Autodesk Inventor part; units mm, degrees
(part 2 of 3)
  line L292 (-4.8745, -39.6988) -> (-5.1074, -39.4176)
  spline S165 degree 2 poles (-5.1074, -39.4176) (-4.9285, -39.2301) (-4.4598, -39) (-4.1502, -39) knots 0 0 0 1 2 2 2
  spline S166 degree 2 poles (-4.1502, -39) (-3.94, -39) (-3.5906, -39.125) (-3.3406, -39.3636) (-3.2014, -39.7073) (-3.2014, -39.9232) knots 0 0 0 1 2 3 4 4 4
  spline S167 degree 2 poles (-3.2014, -39.9232) (-3.2014, -40.1078) (-3.298, -40.4174) (-3.494, -40.7242) (-3.7923, -41.0537) (-3.9968, -41.2525) knots 0 0 0 1 2 3 4 4 4
  line L293 (-3.9968, -41.2525) -> (-4.5706, -41.8121)
  line L294 (-4.5706, -41.8121) -> (-3.031, -41.8121)
  line L295 (-3.031, -41.8121) -> (-3.031, -42.2154)
  spline S168 degree 2 poles (-0.2274, -40.6304) (-0.2274, -40.994) (-0.3723, -41.5934) (-0.6677, -42.0223) (-1.108, -42.2581) (-1.4034, -42.2581) knots 0 0 0 1 2 3 4 4 4
  spline S169 degree 2 poles (-1.4034, -42.2581) (-1.659, -42.2581) (-2.0738, -42.0677) (-2.372, -41.6672) (-2.5311, -41.0537) (-2.5311, -40.6304) knots 0 0 0 1 2 3 4 4 4
  spline S170 degree 2 poles (-2.5311, -40.6304) (-2.5311, -40.2669) (-2.3834, -39.6647) (-2.0908, -39.2358) (-1.6477, -39) (-1.3551, -39) knots 0 0 0 1 2 3 4 4 4
  spline S171 degree 2 poles (-1.3551, -39) (-1.0995, -39) (-0.6819, -39.1903) (-0.3865, -39.5908) (-0.2274, -40.2072) (-0.2274, -40.6304) knots 0 0 0 1 2 3 4 4 4
  spline S172 degree 2 poles (-0.6535, -40.6447) (-0.6535, -40.5623) (-0.6649, -40.4004) (-0.6734, -40.3237) knots 0 0 0 1 2 2 2
  line L296 (-0.6734, -40.3237) -> (-2.0141, -41.3178)
  spline S173 degree 2 poles (-2.0141, -41.3178) (-1.98, -41.4457) (-1.8664, -41.6587) (-1.7102, -41.8121) (-1.5085, -41.8973) (-1.3778, -41.8973) knots 0 0 0 1 2 3 4 4 4
  spline S174 degree 2 poles (-1.3778, -41.8973) (-1.2131, -41.8973) (-0.9461, -41.7382) (-0.7558, -41.4201) (-0.6535, -40.9514) (-0.6535, -40.6447) knots 0 0 0 1 2 3 4 4 4
  spline S175 degree 2 poles (-2.105, -40.6162) (-2.105, -40.6901) (-2.1022, -40.8406) (-2.0965, -40.9117) knots 0 0 0 1 2 2 2
  line L297 (-2.0965, -40.9117) -> (-0.7529, -39.9203)
  spline S176 degree 2 poles (-0.7529, -39.9203) (-0.7899, -39.7953) (-0.9006, -39.5908) (-1.0569, -39.4431) (-1.2557, -39.3607) (-1.3778, -39.3607) knots 0 0 0 1 2 3 4 4 4
  spline S177 degree 2 poles (-1.3778, -39.3607) (-1.5454, -39.3607) (-1.8124, -39.5198) (-2.0028, -39.8379) (-2.105, -40.3066) (-2.105, -40.6162) knots 0 0 0 1 2 3 4 4 4
  line L298 (2.116, -42.2154) -> (2.116, -40.4657)
  spline S178 degree 2 poles (2.116, -40.4657) (2.116, -40.3521) (2.0989, -40.2072) (2.0648, -40.122) (2.0137, -40.0879) (1.974, -40.0879) knots 0 0 0 1 2 3 4 4 4
  spline S179 degree 2 poles (1.974, -40.0879) (1.9285, -40.0879) (1.8518, -40.1447) (1.7638, -40.2782) (1.6587, -40.4941) (1.5848, -40.6503) knots 0 0 0 1 2 3 4 4 4
  line L299 (1.5848, -40.6503) -> (1.5848, -42.2154)
  line L300 (1.5848, -42.2154) -> (1.1616, -42.2154)
  line L301 (1.1616, -42.2154) -> (1.1616, -40.5111)
  spline S180 degree 2 poles (1.1616, -40.5111) (1.1616, -40.3776) (1.1445, -40.2129) (1.1104, -40.122) (1.0565, -40.0879) (1.0167, -40.0879) knots 0 0 0 1 2 3 4 4 4
  spline S181 degree 2 poles (1.0167, -40.0879) (0.9769, -40.0879) (0.9031, -40.1362) (0.815, -40.2612) (0.7042, -40.4799) (0.6304, -40.6503) knots 0 0 0 1 2 3 4 4 4
  line L302 (0.6304, -40.6503) -> (0.6304, -42.2154)
  line L303 (0.6304, -42.2154) -> (0.2072, -42.2154)
  line L304 (0.2072, -42.2154) -> (0.2072, -39.7811)
  line L305 (0.2072, -39.7811) -> (0.5594, -39.7811)
  line L306 (0.5594, -39.7811) -> (0.5793, -40.2441)
  spline S182 degree 2 poles (0.5793, -40.2441) (0.6446, -40.105) (0.7639, -39.9118) (0.8889, -39.7925) (1.0337, -39.7357) (1.119, -39.7357) knots 0 0 0 1 2 3 4 4 4
  spline S183 degree 2 poles (1.119, -39.7357) (1.3178, -39.7357) (1.5223, -39.9942) (1.5223, -40.264) knots 0 0 0 1 2 2 2
  spline S184 degree 2 poles (1.5223, -40.264) (1.5791, -40.1362) (1.6927, -39.9402) (1.8206, -39.8067) (1.9768, -39.7357) (2.0791, -39.7357) knots 0 0 0 1 2 3 4 4 4
  spline S185 degree 2 poles (2.0791, -39.7357) (2.5392, -39.7357) (2.5392, -40.443) knots 0 0 0 1 1 1
  line L307 (2.5392, -40.443) -> (2.5392, -42.2154)
  line L308 (2.5392, -42.2154) -> (2.116, -42.2154)
  line L309 (5.4308, -42.2154) -> (4.9593, -42.2154)
  line L310 (4.9593, -42.2154) -> (4.7406, -41.5252)
  line L311 (4.7406, -41.5252) -> (3.4141, -41.5252)
  line L312 (3.4141, -41.5252) -> (3.1925, -42.2154)
  line L313 (3.1925, -42.2154) -> (2.7466, -42.2154)
  line L314 (2.7466, -42.2154) -> (3.7976, -39.0454)
  line L315 (3.7976, -39.0454) -> (4.3912, -39.0454)
  line L316 (4.3912, -39.0454) -> (5.4308, -42.2154)
  line L317 (4.6156, -41.1389) -> (4.0788, -39.4403)
  line L318 (4.0788, -39.4403) -> (3.5362, -41.1389)
  line L319 (3.5362, -41.1389) -> (4.6156, -41.1389)
  line L320 (-112.276, -39.2585) -> (-113.3553, -42.4285)
  line L321 (-113.3553, -42.4285) -> (-113.9377, -42.4285)
  line L322 (-113.9377, -42.4285) -> (-114.9886, -39.2585)
  line L323 (-114.9886, -39.2585) -> (-114.5029, -39.2585)
  line L324 (-114.5029, -39.2585) -> (-113.8184, -41.3945)
  line L325 (-113.8184, -41.3945) -> (-113.6224, -42.0223)
  line L326 (-113.6224, -42.0223) -> (-113.4235, -41.3945)
  line L327 (-113.4235, -41.3945) -> (-112.739, -39.2585)
  line L328 (-112.739, -39.2585) -> (-112.276, -39.2585)
  spline S186 degree 2 poles (-109.7593, -41.19) (-109.7593, -41.4741) (-109.9183, -41.9484) (-110.2194, -42.2836) (-110.6512, -42.4711) (-110.9267, -42.4711) knots 0 0 0 1 2 3 4 4 4
  spline S187 degree 2 poles (-110.9267, -42.4711) (-111.188, -42.4711) (-111.6028, -42.3092) (-111.8897, -41.9939) (-112.043, -41.528) (-112.043, -41.2241) knots 0 0 0 1 2 3 4 4 4
  spline S188 degree 2 poles (-112.043, -41.2241) (-112.043, -40.9401) (-111.884, -40.4714) (-111.5829, -40.1362) (-111.1511, -39.9487) (-110.8756, -39.9487) knots 0 0 0 1 2 3 4 4 4
  spline S189 degree 2 poles (-110.8756, -39.9487) (-110.6143, -39.9487) (-110.1996, -40.1106) (-109.9127, -40.4231) (-109.7593, -40.8889) (-109.7593, -41.19) knots 0 0 0 1 2 3 4 4 4
  spline S190 degree 2 poles (-110.191, -41.2099) (-110.191, -40.9827) (-110.2904, -40.6475) (-110.4751, -40.4203) (-110.7392, -40.3066) (-110.9012, -40.3066) knots 0 0 0 1 2 3 4 4 4
  spline S191 degree 2 poles (-110.9012, -40.3066) (-111.0915, -40.3066) (-111.3585, -40.4543) (-111.5317, -40.7015) (-111.6113, -41.0281) (-111.6113, -41.2099) knots 0 0 0 1 2 3 4 4 4
  spline S192 degree 2 poles (-111.6113, -41.2099) (-111.6113, -41.4343) (-111.5119, -41.7723) (-111.3272, -41.9996) (-111.0659, -42.1132) (-110.9012, -42.1132) knots 0 0 0 1 2 3 4 4 4
  spline S193 degree 2 poles (-110.9012, -42.1132) (-110.7108, -42.1132) (-110.4438, -41.9655) (-110.2706, -41.7184) (-110.191, -41.3917) (-110.191, -41.2099) knots 0 0 0 1 2 3 4 4 4
  line L329 (-108.3163, -39.3465) -> (-109.0378, -39.3465)
  line L330 (-109.0378, -39.3465) -> (-109.0378, -39)
  line L331 (-109.0378, -39) -> (-107.8902, -39)
  line L332 (-107.8902, -39) -> (-107.8902, -42.0763)
  line L333 (-107.8902, -42.0763) -> (-107.1659, -42.0763)
  line L334 (-107.1659, -42.0763) -> (-107.1659, -42.4285)
  line L335 (-107.1659, -42.4285) -> (-109.1173, -42.4285)
  line L336 (-109.1173, -42.4285) -> (-109.1173, -42.0763)
  line L337 (-109.1173, -42.0763) -> (-108.3163, -42.0763)
  line L338 (-108.3163, -42.0763) -> (-108.3163, -39.3465)
  spline S194 degree 2 poles (-104.4504, -42.3944) (-104.5924, -42.4313) (-104.8992, -42.4626) (-105.0582, -42.4626) knots 0 0 0 1 2 2 2
  spline S195 degree 2 poles (-105.0582, -42.4626) (-105.5156, -42.4626) (-105.9672, -42.0479) (-105.9672, -41.6189) knots 0 0 0 1 2 2 2
  line L339 (-105.9672, -41.6189) -> (-105.9672, -40.3492)
  line L340 (-105.9672, -40.3492) -> (-106.6489, -40.3492)
  line L341 (-106.6489, -40.3492) -> (-106.6489, -39.9942)
  line L342 (-106.6489, -39.9942) -> (-105.9672, -39.9942)
  line L343 (-105.9672, -39.9942) -> (-105.9672, -39.3238)
  line L344 (-105.9672, -39.3238) -> (-105.544, -39.2159)
  line L345 (-105.544, -39.2159) -> (-105.544, -39.9942)
  line L346 (-105.544, -39.9942) -> (-104.4504, -39.9942)
  line L347 (-104.4504, -39.9942) -> (-104.4504, -40.3492)
  line L348 (-104.4504, -40.3492) -> (-105.544, -40.3492)
  line L349 (-105.544, -40.3492) -> (-105.544, -41.5849)
  spline S196 degree 2 poles (-105.544, -41.5849) (-105.544, -41.8462) (-105.2656, -42.1047) (-104.9929, -42.1047) knots 0 0 0 1 2 2 2
  spline S197 degree 2 poles (-104.9929, -42.1047) (-104.8765, -42.1047) (-104.6009, -42.0677) (-104.4504, -42.0308) knots 0 0 0 1 2 2 2
  line L350 (-104.4504, -42.0308) -> (-104.4504, -42.3944)
  line L351 (-101.9422, -42.4285) -> (-101.9422, -40.6787)
  spline S198 degree 2 poles (-101.9422, -40.6787) (-101.9422, -40.5651) (-101.9593, -40.4203) (-101.9933, -40.335) (-102.0445, -40.3009) (-102.0842, -40.3009) knots 0 0 0 1 2 3 4 4 4
  spline S199 degree 2 poles (-102.0842, -40.3009) (-102.1297, -40.3009) (-102.2064, -40.3578) (-102.2944, -40.4913) (-102.3995, -40.7071) (-102.4734, -40.8634) knots 0 0 0 1 2 3 4 4 4
  line L352 (-102.4734, -40.8634) -> (-102.4734, -42.4285)
  line L353 (-102.4734, -42.4285) -> (-102.8966, -42.4285)
  line L354 (-102.8966, -42.4285) -> (-102.8966, -40.7242)
  spline S200 degree 2 poles (-102.8966, -40.7242) (-102.8966, -40.5907) (-102.9137, -40.4259) (-102.9478, -40.335) (-103.0017, -40.3009) (-103.0415, -40.3009) knots 0 0 0 1 2 3 4 4 4
  spline S201 degree 2 poles (-103.0415, -40.3009) (-103.0813, -40.3009) (-103.1551, -40.3492) (-103.2432, -40.4742) (-103.3539, -40.6929) (-103.4278, -40.8634) knots 0 0 0 1 2 3 4 4 4
  line L355 (-103.4278, -40.8634) -> (-103.4278, -42.4285)
  line L356 (-103.4278, -42.4285) -> (-103.851, -42.4285)
  line L357 (-103.851, -42.4285) -> (-103.851, -39.9942)
  line L358 (-103.851, -39.9942) -> (-103.4988, -39.9942)
  line L359 (-103.4988, -39.9942) -> (-103.4789, -40.4572)
  spline S202 degree 2 poles (-103.4789, -40.4572) (-103.4136, -40.318) (-103.2943, -40.1248) (-103.1693, -40.0055) (-103.0244, -39.9487) (-102.9392, -39.9487) knots 0 0 0 1 2 3 4 4 4
  spline S203 degree 2 poles (-102.9392, -39.9487) (-102.7404, -39.9487) (-102.5359, -40.2072) (-102.5359, -40.4771) knots 0 0 0 1 2 2 2
  spline S204 degree 2 poles (-102.5359, -40.4771) (-102.4791, -40.3492) (-102.3654, -40.1532) (-102.2376, -40.0197) (-102.0814, -39.9487) (-101.9791, -39.9487) knots 0 0 0 1 2 3 4 4 4
  spline S205 degree 2 poles (-101.9791, -39.9487) (-101.519, -39.9487) (-101.519, -40.656) knots 0 0 0 1 1 1
  line L360 (-101.519, -40.656) -> (-101.519, -42.4285)
  line L361 (-101.519, -42.4285) -> (-101.9422, -42.4285)
  spline S206 degree 2 poles (-98.8915, -41.0821) (-98.8915, -41.1701) (-98.8972, -41.2923) (-98.9, -41.3463) knots 0 0 0 1 2 2 2
  line L362 (-98.9, -41.3463) -> (-100.6129, -41.3463)
  spline S207 degree 2 poles (-100.6129, -41.3463) (-100.6129, -41.7184) (-100.1953, -42.1189) (-99.8005, -42.1189) knots 0 0 0 1 2 2 2
  spline S208 degree 2 poles (-99.8005, -42.1189) (-99.6954, -42.1189) (-99.4823, -42.1018) (-99.2807, -42.0734) (-99.0989, -42.0365) (-99.0222, -42.0138) knots 0 0 0 1 2 3 4 4 4
  line L363 (-99.0222, -42.0138) -> (-99.0222, -42.3603)
  spline S209 degree 2 poles (-99.0222, -42.3603) (-99.1954, -42.4086) (-99.63, -42.4711) (-99.863, -42.4711) knots 0 0 0 1 2 2 2
  spline S210 degree 2 poles (-99.863, -42.4711) (-100.1754, -42.4711) (-100.6271, -42.3007) (-100.914, -41.9797) (-101.0531, -41.511) (-101.0531, -41.2156) knots 0 0 0 1 2 3 4 4 4
  spline S211 degree 2 poles (-101.0531, -41.2156) (-101.0531, -40.9571) (-100.9054, -40.4998) (-100.6214, -40.1532) (-100.2095, -39.9487) (-99.9482, -39.9487) knots 0 0 0 1 2 3 4 4 4
  spline S212 degree 2 poles (-99.9482, -39.9487) (-99.6925, -39.9487) (-99.2977, -40.1078) (-99.0307, -40.4032) (-98.8915, -40.8208) (-98.8915, -41.0821) knots 0 0 0 1 2 3 4 4 4
  spline S213 degree 2 poles (-99.3318, -41.0224) (-99.3233, -40.8605) (-99.4028, -40.5907) (-99.5647, -40.3947) (-99.8062, -40.2867) (-99.9681, -40.2867) knots 0 0 0 1 2 3 4 4 4
  spline S214 degree 2 poles (-99.9681, -40.2867) (-100.1044, -40.2867) (-100.3345, -40.3947) (-100.4992, -40.5878) (-100.6015, -40.8605) (-100.6129, -41.0224) knots 0 0 0 1 2 3 4 4 4
  line L364 (-100.6129, -41.0224) -> (-99.3318, -41.0224)
  spline S215 degree 2 poles (-96.2527, -42.3944) (-96.3947, -42.4313) (-96.7015, -42.4626) (-96.8606, -42.4626) knots 0 0 0 1 2 2 2
  spline S216 degree 2 poles (-96.8606, -42.4626) (-97.3179, -42.4626) (-97.7695, -42.0479) (-97.7695, -41.6189) knots 0 0 0 1 2 2 2
  line L365 (-97.7695, -41.6189) -> (-97.7695, -40.3492)
  line L366 (-97.7695, -40.3492) -> (-98.4512, -40.3492)
  line L367 (-98.4512, -40.3492) -> (-98.4512, -39.9942)
  line L368 (-98.4512, -39.9942) -> (-97.7695, -39.9942)
  line L369 (-97.7695, -39.9942) -> (-97.7695, -39.3238)
  line L370 (-97.7695, -39.3238) -> (-97.3463, -39.2159)
  line L371 (-97.3463, -39.2159) -> (-97.3463, -39.9942)
  line L372 (-97.3463, -39.9942) -> (-96.2527, -39.9942)
  line L373 (-96.2527, -39.9942) -> (-96.2527, -40.3492)
  line L374 (-96.2527, -40.3492) -> (-97.3463, -40.3492)
  line L375 (-97.3463, -40.3492) -> (-97.3463, -41.5849)
  spline S217 degree 2 poles (-97.3463, -41.5849) (-97.3463, -41.8462) (-97.0679, -42.1047) (-96.7952, -42.1047) knots 0 0 0 1 2 2 2
  spline S218 degree 2 poles (-96.7952, -42.1047) (-96.6788, -42.1047) (-96.4032, -42.0677) (-96.2527, -42.0308) knots 0 0 0 1 2 2 2
  line L376 (-96.2527, -42.0308) -> (-96.2527, -42.3944)
  spline S219 degree 2 poles (-93.4264, -41.0821) (-93.4264, -41.1701) (-93.4321, -41.2923) (-93.4349, -41.3463) knots 0 0 0 1 2 2 2
  line L377 (-93.4349, -41.3463) -> (-95.1477, -41.3463)
  spline S220 degree 2 poles (-95.1477, -41.3463) (-95.1477, -41.7184) (-94.7302, -42.1189) (-94.3353, -42.1189) knots 0 0 0 1 2 2 2
  spline S221 degree 2 poles (-94.3353, -42.1189) (-94.2303, -42.1189) (-94.0172, -42.1018) (-93.8155, -42.0734) (-93.6337, -42.0365) (-93.5571, -42.0138) knots 0 0 0 1 2 3 4 4 4
  line L378 (-93.5571, -42.0138) -> (-93.5571, -42.3603)
  spline S222 degree 2 poles (-93.5571, -42.3603) (-93.7303, -42.4086) (-94.1649, -42.4711) (-94.3978, -42.4711) knots 0 0 0 1 2 2 2
  spline S223 degree 2 poles (-94.3978, -42.4711) (-94.7103, -42.4711) (-95.1619, -42.3007) (-95.4488, -41.9797) (-95.588, -41.511) (-95.588, -41.2156) knots 0 0 0 1 2 3 4 4 4
  spline S224 degree 2 poles (-95.588, -41.2156) (-95.588, -40.9571) (-95.4403, -40.4998) (-95.1563, -40.1532) (-94.7444, -39.9487) (-94.4831, -39.9487) knots 0 0 0 1 2 3 4 4 4
  spline S225 degree 2 poles (-94.4831, -39.9487) (-94.2274, -39.9487) (-93.8326, -40.1078) (-93.5656, -40.4032) (-93.4264, -40.8208) (-93.4264, -41.0821) knots 0 0 0 1 2 3 4 4 4
  spline S226 degree 2 poles (-93.8667, -41.0224) (-93.8581, -40.8605) (-93.9377, -40.5907) (-94.0996, -40.3947) (-94.341, -40.2867) (-94.5029, -40.2867) knots 0 0 0 1 2 3 4 4 4
  spline S227 degree 2 poles (-94.5029, -40.2867) (-94.6393, -40.2867) (-94.8694, -40.3947) (-95.0341, -40.5878) (-95.1364, -40.8605) (-95.1477, -41.0224) knots 0 0 0 1 2 3 4 4 4
  line L379 (-95.1477, -41.0224) -> (-93.8667, -41.0224)
  line L380 (-92.6509, -39.9942) -> (-92.2646, -39.9942)
  line L381 (-92.2646, -39.9942) -> (-92.2533, -40.443)
  spline S228 degree 2 poles (-92.2533, -40.443) (-92.0374, -40.1816) (-91.6198, -39.9487) (-91.404, -39.9487) knots 0 0 0 1 2 2 2
  spline S229 degree 2 poles (-91.404, -39.9487) (-91.0262, -39.9487) (-90.637, -40.4401) (-90.6512, -40.923) knots 0 0 0 1 2 2 2
  line L382 (-90.6512, -40.923) -> (-91.0773, -40.923)
  spline S230 degree 2 poles (-91.0773, -40.923) (-91.0688, -40.602) (-91.2704, -40.3123) (-91.4664, -40.3123) knots 0 0 0 1 2 2 2
  spline S231 degree 2 poles (-91.4664, -40.3123) (-91.5517, -40.3123) (-91.7221, -40.372) (-91.9039, -40.5083) (-92.1084, -40.7157) (-92.2249, -40.8662) knots 0 0 0 1 2 3 4 4 4
  line L383 (-92.2249, -40.8662) -> (-92.2249, -42.4285)
  line L384 (-92.2249, -42.4285) -> (-92.6509, -42.4285)
  line L385 (-92.6509, -42.4285) -> (-92.6509, -39.9942)
  spline S232 degree 2 poles (-85.1577, -40.8435) (-85.1577, -41.2071) (-85.3026, -41.8064) (-85.598, -42.2353) (-86.0382, -42.4711) (-86.3337, -42.4711) knots 0 0 0 1 2 3 4 4 4
  spline S233 degree 2 poles (-86.3337, -42.4711) (-86.5893, -42.4711) (-87.004, -42.2808) (-87.3023, -41.8803) (-87.4613, -41.2667) (-87.4613, -40.8435) knots 0 0 0 1 2 3 4 4 4
  spline S234 degree 2 poles (-87.4613, -40.8435) (-87.4613, -40.4799) (-87.3136, -39.8777) (-87.0211, -39.4488) (-86.5779, -39.213) (-86.2854, -39.213) knots 0 0 0 1 2 3 4 4 4
  spline S235 degree 2 poles (-86.2854, -39.213) (-86.0297, -39.213) (-85.6122, -39.4034) (-85.3168, -39.8039) (-85.1577, -40.4203) (-85.1577, -40.8435) knots 0 0 0 1 2 3 4 4 4
  spline S236 degree 2 poles (-85.5838, -40.8577) (-85.5838, -40.7753) (-85.5951, -40.6134) (-85.6036, -40.5367) knots 0 0 0 1 2 2 2
  line L386 (-85.6036, -40.5367) -> (-86.9444, -41.5309)
  spline S237 degree 2 poles (-86.9444, -41.5309) (-86.9103, -41.6587) (-86.7967, -41.8717) (-86.6404, -42.0251) (-86.4388, -42.1103) (-86.3081, -42.1103) knots 0 0 0 1 2 3 4 4 4
  spline S238 degree 2 poles (-86.3081, -42.1103) (-86.1433, -42.1103) (-85.8763, -41.9513) (-85.686, -41.6331) (-85.5838, -41.1645) (-85.5838, -40.8577) knots 0 0 0 1 2 3 4 4 4
  spline S239 degree 2 poles (-87.0353, -40.8293) (-87.0353, -40.9031) (-87.0324, -41.0537) (-87.0267, -41.1247) knots 0 0 0 1 2 2 2
  line L387 (-87.0267, -41.1247) -> (-85.6832, -40.1334)
  spline S240 degree 2 poles (-85.6832, -40.1334) (-85.7201, -40.0084) (-85.8309, -39.8039) (-85.9871, -39.6562) (-86.1859, -39.5738) (-86.3081, -39.5738) knots 0 0 0 1 2 3 4 4 4
  spline S241 degree 2 poles (-86.3081, -39.5738) (-86.4757, -39.5738) (-86.7427, -39.7328) (-86.933, -40.051) (-87.0353, -40.5197) (-87.0353, -40.8293) knots 0 0 0 1 2 3 4 4 4
  line L388 (-80.1186, -41.3065) -> (-81.5701, -41.3065)
  line L389 (-81.5701, -41.3065) -> (-81.5701, -40.9088)
  line L390 (-81.5701, -40.9088) -> (-80.1186, -40.9088)
  line L391 (-80.1186, -40.9088) -> (-80.1186, -41.3065)
  line L392 (-74.3269, -42.4285) -> (-76.318, -42.4285)
  line L393 (-76.318, -42.4285) -> (-76.318, -42.0365)
  line L394 (-76.318, -42.0365) -> (-75.5028, -42.0365)
  line L395 (-75.5028, -42.0365) -> (-75.5028, -39.7215)
  line L396 (-75.5028, -39.7215) -> (-76.2612, -40.1334)
  line L397 (-76.2612, -40.1334) -> (-76.4175, -39.7755)
  line L398 (-76.4175, -39.7755) -> (-75.4091, -39.2443)
  line L399 (-75.4091, -39.2443) -> (-75.0341, -39.2443)
  line L400 (-75.0341, -39.2443) -> (-75.0341, -42.0365)
  line L401 (-75.0341, -42.0365) -> (-74.3269, -42.0365)
  line L402 (-74.3269, -42.0365) -> (-74.3269, -42.4285)
  spline S242 degree 2 poles (-71.4949, -40.8435) (-71.4949, -41.2071) (-71.6397, -41.8064) (-71.9352, -42.2353) (-72.3754, -42.4711) (-72.6708, -42.4711) knots 0 0 0 1 2 3 4 4 4
  spline S243 degree 2 poles (-72.6708, -42.4711) (-72.9265, -42.4711) (-73.3412, -42.2808) (-73.6395, -41.8803) (-73.7985, -41.2667) (-73.7985, -40.8435) knots 0 0 0 1 2 3 4 4 4
  spline S244 degree 2 poles (-73.7985, -40.8435) (-73.7985, -40.4799) (-73.6508, -39.8777) (-73.3582, -39.4488) (-72.9151, -39.213) (-72.6226, -39.213) knots 0 0 0 1 2 3 4 4 4
  spline S245 degree 2 poles (-72.6226, -39.213) (-72.3669, -39.213) (-71.9494, -39.4034) (-71.6539, -39.8039) (-71.4949, -40.4203) (-71.4949, -40.8435) knots 0 0 0 1 2 3 4 4 4
  spline S246 degree 2 poles (-71.9209, -40.8577) (-71.9209, -40.7753) (-71.9323, -40.6134) (-71.9408, -40.5367) knots 0 0 0 1 2 2 2
  line L403 (-71.9408, -40.5367) -> (-73.2815, -41.5309)
  spline S247 degree 2 poles (-73.2815, -41.5309) (-73.2475, -41.6587) (-73.1338, -41.8717) (-72.9776, -42.0251) (-72.7759, -42.1103) (-72.6453, -42.1103) knots 0 0 0 1 2 3 4 4 4
  spline S248 degree 2 poles (-72.6453, -42.1103) (-72.4805, -42.1103) (-72.2135, -41.9513) (-72.0232, -41.6331) (-71.9209, -41.1645) (-71.9209, -40.8577) knots 0 0 0 1 2 3 4 4 4
  spline S249 degree 2 poles (-73.3724, -40.8293) (-73.3724, -40.9031) (-73.3696, -41.0537) (-73.3639, -41.1247) knots 0 0 0 1 2 2 2
  line L404 (-73.3639, -41.1247) -> (-72.0204, -40.1334)
  spline S250 degree 2 poles (-72.0204, -40.1334) (-72.0573, -40.0084) (-72.1681, -39.8039) (-72.3243, -39.6562) (-72.5231, -39.5738) (-72.6453, -39.5738) knots 0 0 0 1 2 3 4 4 4
  spline S251 degree 2 poles (-72.6453, -39.5738) (-72.8129, -39.5738) (-73.0799, -39.7328) (-73.2702, -40.051) (-73.3724, -40.5197) (-73.3724, -40.8293) knots 0 0 0 1 2 3 4 4 4
  line L405 (-71.1142, -39.9942) -> (-70.6342, -39.9942)
  line L406 (-70.6342, -39.9942) -> (-70.0405, -41.6047)
  line L407 (-70.0405, -41.6047) -> (-69.9099, -41.9996)
  line L408 (-69.9099, -41.9996) -> (-69.7792, -41.5962)
  line L409 (-69.7792, -41.5962) -> (-69.1884, -39.9942)
  line L410 (-69.1884, -39.9942) -> (-68.7225, -39.9942)
  line L411 (-68.7225, -39.9942) -> (-69.6798, -42.4285)
  line L412 (-69.6798, -42.4285) -> (-70.1627, -42.4285)
  line L413 (-70.1627, -42.4285) -> (-71.1142, -39.9942)
  spline S252 degree 2 poles (21.5536, -6.5964) (21.5536, -6.8236) (21.4826, -7.2412) (21.3292, -7.5991) (21.0821, -7.8916) (20.7213, -8.1018) (20.247, -8.2154) (19.943, -8.2154) knots 0 0 0 1 2 3 4 5 6 6 6
  line L414 (19.943, -8.2154) -> (19.2642, -8.2154)
  line L415 (19.2642, -8.2154) -> (19.2642, -5.0454)
  line L416 (19.2642, -5.0454) -> (20.0822, -5.0454)
  spline S253 degree 2 poles (20.0822, -5.0454) (20.8236, -5.0454) (21.5536, -5.8095) (21.5536, -6.5964) knots 0 0 0 1 2 2 2
  spline S254 degree 2 poles (21.0991, -6.6248) (21.0991, -6.2896) (20.9741, -5.8237) (20.7157, -5.5369) (20.3294, -5.409) (20.068, -5.409) knots 0 0 0 1 2 3 4 4 4
  line L417 (20.068, -5.409) -> (19.6959, -5.409)
  line L418 (19.6959, -5.409) -> (19.6959, -7.8405)
  line L419 (19.6959, -7.8405) -> (20.0169, -7.8405)
  spline S255 degree 2 poles (20.0169, -7.8405) (21.0991, -7.8405) (21.0991, -6.6248) knots 0 0 0 1 1 1
  spline S256 degree 2 poles (24.3316, -6.6077) (24.3316, -7.0366) (24.1299, -7.6559) (23.7891, -8.0621) (23.3289, -8.2581) (23.0761, -8.2581) knots 0 0 0 1 2 3 4 4 4
  spline S257 degree 2 poles (23.0761, -8.2581) (22.7693, -8.2581) (22.3149, -8.0365) (22.0166, -7.6189) (21.8717, -7.0196) (21.8717, -6.6447) knots 0 0 0 1 2 3 4 4 4
  spline S258 degree 2 poles (21.8717, -6.6447) (21.8717, -6.2214) (22.0706, -5.6022) (22.4114, -5.196) (22.8688, -5) (23.1244, -5) knots 0 0 0 1 2 3 4 4 4
  spline S259 degree 2 poles (23.1244, -5) (23.4283, -5) (23.8828, -5.2244) (24.1839, -5.6391) (24.3316, -6.2356) (24.3316, -6.6077) knots 0 0 0 1 2 3 4 4 4
  spline S260 degree 2 poles (23.8999, -6.639) (23.8999, -6.3606) (23.8118, -5.8976) (23.6187, -5.5624) (23.3147, -5.3778) (23.0988, -5.3778) knots 0 0 0 1 2 3 4 4 4
  spline S261 degree 2 poles (23.0988, -5.3778) (22.8915, -5.3778) (22.5904, -5.5738) (22.3972, -5.9118) (22.3035, -6.3663) (22.3035, -6.6219) knots 0 0 0 1 2 3 4 4 4
  spline S262 degree 2 poles (22.3035, -6.6219) (22.3035, -6.9031) (22.3916, -7.3661) (22.5847, -7.6985) (22.8858, -7.8831) (23.0988, -7.8831) knots 0 0 0 1 2 3 4 4 4
  spline S263 degree 2 poles (23.0988, -7.8831) (23.3062, -7.8831) (23.6101, -7.6871) (23.8061, -7.3491) (23.8999, -6.8975) (23.8999, -6.639) knots 0 0 0 1 2 3 4 4 4
  spline S264 degree 2 poles (29.5809, -7.2525) (29.5809, -7.4599) (29.4104, -7.8263) (29.0724, -8.1018) (28.5583, -8.2581) (28.2146, -8.2581) knots 0 0 0 1 2 3 4 4 4
  spline S265 degree 2 poles (28.2146, -8.2581) (28.0271, -8.2581) (27.726, -8.2325) (27.5954, -8.2126) knots 0 0 0 1 2 2 2
  line L420 (27.5954, -8.2126) -> (27.5954, -7.8348)
  spline S266 degree 2 poles (27.5954, -7.8348) (27.7459, -7.8632) (28.0811, -7.8916) (28.2544, -7.8916) knots 0 0 0 1 2 2 2
  spline S267 degree 2 poles (28.2544, -7.8916) (28.493, -7.8916) (28.831, -7.8064) (29.044, -7.6473) (29.1406, -7.4201) (29.1406, -7.2781) knots 0 0 0 1 2 3 4 4 4
  spline S268 degree 2 poles (29.1406, -7.2781) (29.1406, -7.1446) (29.0241, -6.9514) (28.8139, -6.8208) (28.5214, -6.7554) (28.3453, -6.7554) knots 0 0 0 1 2 3 4 4 4
  line L421 (28.3453, -6.7554) -> (27.9845, -6.7554)
  line L422 (27.9845, -6.7554) -> (27.9845, -6.4089)
  line L423 (27.9845, -6.4089) -> (28.3509, -6.4089)
  spline S269 degree 2 poles (28.3509, -6.4089) (28.493, -6.4089) (28.7287, -6.3322) (28.8935, -6.193) (28.9844, -5.9857) (28.9844, -5.855) knots 0 0 0 1 2 3 4 4 4
  spline S270 degree 2 poles (28.9844, -5.855) (28.9844, -5.5993) (28.6747, -5.3664) (28.3737, -5.3664) knots 0 0 0 1 2 2 2
  spline S271 degree 2 poles (28.3737, -5.3664) (28.2146, -5.3664) (27.8737, -5.4289) (27.6806, -5.4914) knots 0 0 0 1 2 2 2
  line L424 (27.6806, -5.4914) -> (27.6806, -5.1221)
  spline S272 degree 2 poles (27.6806, -5.1221) (27.7629, -5.0937) (27.9504, -5.0483) (28.1351, -5.017) (28.3197, -5) (28.4049, -5) knots 0 0 0 1 2 3 4 4 4
  spline S273 degree 2 poles (28.4049, -5) (28.6577, -5) (29.0412, -5.1079) (29.2968, -5.3125) (29.4275, -5.605) (29.4275, -5.7868) knots 0 0 0 1 2 3 4 4 4
  spline S274 degree 2 poles (29.4275, -5.7868) (29.4275, -6.0595) (29.1491, -6.4288) (28.9077, -6.5367) knots 0 0 0 1 2 2 2
  spline S275 degree 2 poles (28.9077, -6.5367) (29.0298, -6.5566) (29.2713, -6.6731) (29.4616, -6.8548) (29.5809, -7.102) (29.5809, -7.2525) knots 0 0 0 1 2 3 4 4 4
  spline S276 degree 2 poles (21.5536, 18.4036) (21.5536, 18.1764) (21.4826, 17.7588) (21.3292, 17.4009) (21.0821, 17.1084) (20.7213, 16.8982) (20.247, 16.7846) (19.943, 16.7846) knots 0 0 0 1 2 3 4 5 6 6 6
  line L425 (19.943, 16.7846) -> (19.2642, 16.7846)
  line L426 (19.2642, 16.7846) -> (19.2642, 19.9546)
  line L427 (19.2642, 19.9546) -> (20.0822, 19.9546)
  spline S277 degree 2 poles (20.0822, 19.9546) (20.8236, 19.9546) (21.5536, 19.1905) (21.5536, 18.4036) knots 0 0 0 1 2 2 2
  spline S278 degree 2 poles (21.0991, 18.3752) (21.0991, 18.7104) (20.9741, 19.1763) (20.7157, 19.4631) (20.3294, 19.591) (20.068, 19.591) knots 0 0 0 1 2 3 4 4 4
  line L428 (20.068, 19.591) -> (19.6959, 19.591)
  line L429 (19.6959, 19.591) -> (19.6959, 17.1595)
  line L430 (19.6959, 17.1595) -> (20.0169, 17.1595)
  spline S279 degree 2 poles (20.0169, 17.1595) (21.0991, 17.1595) (21.0991, 18.3752) knots 0 0 0 1 1 1
  spline S280 degree 2 poles (24.3316, 18.3923) (24.3316, 17.9634) (24.1299, 17.3441) (23.7891, 16.9379) (23.3289, 16.7419) (23.0761, 16.7419) knots 0 0 0 1 2 3 4 4 4
  spline S281 degree 2 poles (23.0761, 16.7419) (22.7693, 16.7419) (22.3149, 16.9635) (22.0166, 17.3811) (21.8717, 17.9804) (21.8717, 18.3553) knots 0 0 0 1 2 3 4 4 4
  spline S282 degree 2 poles (21.8717, 18.3553) (21.8717, 18.7786) (22.0706, 19.3978) (22.4114, 19.804) (22.8688, 20) (23.1244, 20) knots 0 0 0 1 2 3 4 4 4
  spline S283 degree 2 poles (23.1244, 20) (23.4283, 20) (23.8828, 19.7756) (24.1839, 19.3609) (24.3316, 18.7644) (24.3316, 18.3923) knots 0 0 0 1 2 3 4 4 4
  spline S284 degree 2 poles (23.8999, 18.361) (23.8999, 18.6394) (23.8118, 19.1024) (23.6187, 19.4376) (23.3147, 19.6222) (23.0988, 19.6222) knots 0 0 0 1 2 3 4 4 4
  spline S285 degree 2 poles (23.0988, 19.6222) (22.8915, 19.6222) (22.5904, 19.4262) (22.3972, 19.0882) (22.3035, 18.6337) (22.3035, 18.3781) knots 0 0 0 1 2 3 4 4 4
  spline S286 degree 2 poles (22.3035, 18.3781) (22.3035, 18.0969) (22.3916, 17.6339) (22.5847, 17.3015) (22.8858, 17.1169) (23.0988, 17.1169) knots 0 0 0 1 2 3 4 4 4
  spline S287 degree 2 poles (23.0988, 17.1169) (23.3062, 17.1169) (23.6101, 17.3129) (23.8061, 17.6509) (23.8999, 18.1025) (23.8999, 18.361) knots 0 0 0 1 2 3 4 4 4
  line L431 (29.615, 16.7846) -> (27.6238, 16.7846)
  line L432 (27.6238, 16.7846) -> (27.6238, 17.1765)
  line L433 (27.6238, 17.1765) -> (28.439, 17.1765)
  line L434 (28.439, 17.1765) -> (28.439, 19.4916)
  line L435 (28.439, 19.4916) -> (27.6806, 19.0797)
  line L436 (27.6806, 19.0797) -> (27.5243, 19.4376)
  line L437 (27.5243, 19.4376) -> (28.5327, 19.9688)
  line L438 (28.5327, 19.9688) -> (28.9077, 19.9688)
  line L439 (28.9077, 19.9688) -> (28.9077, 17.1765)
  line L440 (28.9077, 17.1765) -> (29.615, 17.1765)
  line L441 (29.615, 17.1765) -> (29.615, 16.7846)
  spline S288 degree 2 poles (41.5536, 18.4036) (41.5536, 18.1764) (41.4826, 17.7588) (41.3292, 17.4009) (41.0821, 17.1084) (40.7213, 16.8982) (40.247, 16.7846) (39.943, 16.7846) knots 0 0 0 1 2 3 4 5 6 6 6
  line L442 (39.943, 16.7846) -> (39.2642, 16.7846)
  line L443 (39.2642, 16.7846) -> (39.2642, 19.9546)
  line L444 (39.2642, 19.9546) -> (40.0822, 19.9546)
  spline S289 degree 2 poles (40.0822, 19.9546) (40.8236, 19.9546) (41.5536, 19.1905) (41.5536, 18.4036) knots 0 0 0 1 2 2 2
  spline S290 degree 2 poles (41.0991, 18.3752) (41.0991, 18.7104) (40.9741, 19.1763) (40.7157, 19.4631) (40.3294, 19.591) (40.068, 19.591) knots 0 0 0 1 2 3 4 4 4
  line L445 (40.068, 19.591) -> (39.6959, 19.591)
  line L446 (39.6959, 19.591) -> (39.6959, 17.1595)
  line L447 (39.6959, 17.1595) -> (40.0169, 17.1595)
  spline S291 degree 2 poles (40.0169, 17.1595) (41.0991, 17.1595) (41.0991, 18.3752) knots 0 0 0 1 1 1
  spline S292 degree 2 poles (44.3316, 18.3923) (44.3316, 17.9634) (44.1299, 17.3441) (43.7891, 16.9379) (43.3289, 16.7419) (43.0761, 16.7419) knots 0 0 0 1 2 3 4 4 4
  spline S293 degree 2 poles (43.0761, 16.7419) (42.7693, 16.7419) (42.3149, 16.9635) (42.0166, 17.3811) (41.8717, 17.9804) (41.8717, 18.3553) knots 0 0 0 1 2 3 4 4 4
  spline S294 degree 2 poles (41.8717, 18.3553) (41.8717, 18.7786) (42.0706, 19.3978) (42.4114, 19.804) (42.8688, 20) (43.1244, 20) knots 0 0 0 1 2 3 4 4 4
  spline S295 degree 2 poles (43.1244, 20) (43.4283, 20) (43.8828, 19.7756) (44.1839, 19.3609) (44.3316, 18.7644) (44.3316, 18.3923) knots 0 0 0 1 2 3 4 4 4
  spline S296 degree 2 poles (43.8999, 18.361) (43.8999, 18.6394) (43.8118, 19.1024) (43.6187, 19.4376) (43.3147, 19.6222) (43.0988, 19.6222) knots 0 0 0 1 2 3 4 4 4
  spline S297 degree 2 poles (43.0988, 19.6222) (42.8915, 19.6222) (42.5904, 19.4262) (42.3972, 19.0882) (42.3035, 18.6337) (42.3035, 18.3781) knots 0 0 0 1 2 3 4 4 4
  spline S298 degree 2 poles (42.3035, 18.3781) (42.3035, 18.0969) (42.3916, 17.6339) (42.5847, 17.3015) (42.8858, 17.1169) (43.0988, 17.1169) knots 0 0 0 1 2 3 4 4 4
  spline S299 degree 2 poles (43.0988, 17.1169) (43.3062, 17.1169) (43.6101, 17.3129) (43.8061, 17.6509) (43.8999, 18.1025) (43.8999, 18.361) knots 0 0 0 1 2 3 4 4 4
  line L448 (49.6434, 16.7846) -> (47.5556, 16.7846)
  line L449 (47.5556, 16.7846) -> (47.5556, 17.1623)
  line L450 (47.5556, 17.1623) -> (48.3737, 17.9776)
  spline S300 degree 2 poles (48.3737, 17.9776) (48.5753, 18.1764) (48.8281, 18.469) (48.9673, 18.7104) (49.0156, 18.9234) (49.0156, 19.0456) knots 0 0 0 1 2 3 4 4 4
  spline S301 degree 2 poles (49.0156, 19.0456) (49.0156, 19.1621) (48.9531, 19.3722) (48.8225, 19.5342) (48.6123, 19.6251) (48.4674, 19.6251) knots 0 0 0 1 2 3 4 4 4
  spline S302 degree 2 poles (48.4674, 19.6251) (48.2657, 19.6251) (47.9362, 19.4461) (47.7999, 19.3012) knots 0 0 0 1 2 2 2
  line L451 (47.7999, 19.3012) -> (47.567, 19.5824)
  spline S303 degree 2 poles (47.567, 19.5824) (47.7459, 19.7699) (48.2146, 20) (48.5242, 20) knots 0 0 0 1 2 2 2
  spline S304 degree 2 poles (48.5242, 20) (48.7344, 20) (49.0838, 19.875) (49.3337, 19.6364) (49.4729, 19.2927) (49.4729, 19.0768) knots 0 0 0 1 2 3 4 4 4
  spline S305 degree 2 poles (49.4729, 19.0768) (49.4729, 18.8922) (49.3764, 18.5826) (49.1804, 18.2758) (48.8821, 17.9463) (48.6776, 17.7475) knots 0 0 0 1 2 3 4 4 4
  line L452 (48.6776, 17.7475) -> (48.1038, 17.1879)
  line L453 (48.1038, 17.1879) -> (49.6434, 17.1879)
  line L454 (49.6434, 17.1879) -> (49.6434, 16.7846)
  spline S306 degree 2 poles (41.5536, -6.5964) (41.5536, -6.8236) (41.4826, -7.2412) (41.3292, -7.5991) (41.0821, -7.8916) (40.7213, -8.1018) (40.247, -8.2154) (39.943, -8.2154) knots 0 0 0 1 2 3 4 5 6 6 6
  line L455 (39.943, -8.2154) -> (39.2642, -8.2154)
  line L456 (39.2642, -8.2154) -> (39.2642, -5.0454)
  line L457 (39.2642, -5.0454) -> (40.0822, -5.0454)
  spline S307 degree 2 poles (40.0822, -5.0454) (40.8236, -5.0454) (41.5536, -5.8095) (41.5536, -6.5964) knots 0 0 0 1 2 2 2
  spline S308 degree 2 poles (41.0991, -6.6248) (41.0991, -6.2896) (40.9741, -5.8237) (40.7157, -5.5369) (40.3294, -5.409) (40.068, -5.409) knots 0 0 0 1 2 3 4 4 4
  line L458 (40.068, -5.409) -> (39.6959, -5.409)
  line L459 (39.6959, -5.409) -> (39.6959, -7.8405)
  line L460 (39.6959, -7.8405) -> (40.0169, -7.8405)
  spline S309 degree 2 poles (40.0169, -7.8405) (41.0991, -7.8405) (41.0991, -6.6248) knots 0 0 0 1 1 1
  spline S310 degree 2 poles (44.3316, -6.6077) (44.3316, -7.0366) (44.1299, -7.6559) (43.7891, -8.0621) (43.3289, -8.2581) (43.0761, -8.2581) knots 0 0 0 1 2 3 4 4 4
  spline S311 degree 2 poles (43.0761, -8.2581) (42.7693, -8.2581) (42.3149, -8.0365) (42.0166, -7.6189) (41.8717, -7.0196) (41.8717, -6.6447) knots 0 0 0 1 2 3 4 4 4
  spline S312 degree 2 poles (41.8717, -6.6447) (41.8717, -6.2214) (42.0706, -5.6022) (42.4114, -5.196) (42.8688, -5) (43.1244, -5) knots 0 0 0 1 2 3 4 4 4
  spline S313 degree 2 poles (43.1244, -5) (43.4283, -5) (43.8828, -5.2244) (44.1839, -5.6391) (44.3316, -6.2356) (44.3316, -6.6077) knots 0 0 0 1 2 3 4 4 4
  spline S314 degree 2 poles (43.8999, -6.639) (43.8999, -6.3606) (43.8118, -5.8976) (43.6187, -5.5624) (43.3147, -5.3778) (43.0988, -5.3778) knots 0 0 0 1 2 3 4 4 4
  spline S315 degree 2 poles (43.0988, -5.3778) (42.8915, -5.3778) (42.5904, -5.5738) (42.3972, -5.9118) (42.3035, -6.3663) (42.3035, -6.6219) knots 0 0 0 1 2 3 4 4 4
  spline S316 degree 2 poles (42.3035, -6.6219) (42.3035, -6.9031) (42.3916, -7.3661) (42.5847, -7.6985) (42.8858, -7.8831) (43.0988, -7.8831) knots 0 0 0 1 2 3 4 4 4
  spline S317 degree 2 poles (43.0988, -7.8831) (43.3062, -7.8831) (43.6101, -7.6871) (43.8061, -7.3491) (43.8999, -6.8975) (43.8999, -6.639) knots 0 0 0 1 2 3 4 4 4
  line L461 (49.8024, -7.5138) -> (49.2599, -7.5138)
  line L462 (49.2599, -7.5138) -> (49.2599, -8.2154)
  line L463 (49.2599, -8.2154) -> (48.8281, -8.2154)
  line L464 (48.8281, -8.2154) -> (48.8281, -7.5138)
  line L465 (48.8281, -7.5138) -> (47.3028, -7.5138)
  line L466 (47.3028, -7.5138) -> (47.3028, -7.1417)
  line L467 (47.3028, -7.1417) -> (48.6549, -5.0454)
  line L468 (48.6549, -5.0454) -> (49.2599, -5.0454)
  line L469 (49.2599, -5.0454) -> (49.2599, -7.1417)
  line L470 (49.2599, -7.1417) -> (49.8024, -7.1417)
  line L471 (49.8024, -7.1417) -> (49.8024, -7.5138)
  line L472 (48.8281, -5.4516) -> (47.726, -7.1417)
  line L473 (47.726, -7.1417) -> (48.8281, -7.1417)
  line L474 (48.8281, -7.1417) -> (48.8281, -5.4516)
  line L475 (75.7098, 16.8158) -> (75.2383, 16.8158)
  line L476 (75.2383, 16.8158) -> (75.0196, 17.506)
  line L477 (75.0196, 17.506) -> (73.6931, 17.506)
  line L478 (73.6931, 17.506) -> (73.4715, 16.8158)
  line L479 (73.4715, 16.8158) -> (73.0256, 16.8158)
  line L480 (73.0256, 16.8158) -> (74.0766, 19.9858)
  line L481 (74.0766, 19.9858) -> (74.6702, 19.9858)
  line L482 (74.6702, 19.9858) -> (75.7098, 16.8158)
  line L483 (74.8946, 17.8923) -> (74.3578, 19.591)
  line L484 (74.3578, 19.591) -> (73.8152, 17.8923)
  line L485 (73.8152, 17.8923) -> (74.8946, 17.8923)
  line L486 (76.8801, 19.6222) -> (76.1501, 19.6222)
  line L487 (76.1501, 19.6222) -> (76.1501, 19.9858)
  line L488 (76.1501, 19.9858) -> (78.0476, 19.9858)
  line L489 (78.0476, 19.9858) -> (78.0476, 19.6222)
  line L490 (78.0476, 19.6222) -> (77.3176, 19.6222)
  line L491 (77.3176, 19.6222) -> (77.3176, 17.1851)
  line L492 (77.3176, 17.1851) -> (78.0476, 17.1851)
  line L493 (78.0476, 17.1851) -> (78.0476, 16.8158)
  line L494 (78.0476, 16.8158) -> (76.1501, 16.8158)
  line L495 (76.1501, 16.8158) -> (76.1501, 17.1851)
  line L496 (76.1501, 17.1851) -> (76.8801, 17.1851)
  line L497 (76.8801, 17.1851) -> (76.8801, 19.6222)
  line L498 (83.615, 16.8158) -> (81.6238, 16.8158)
  line L499 (81.6238, 16.8158) -> (81.6238, 17.2078)
  line L500 (81.6238, 17.2078) -> (82.439, 17.2078)
  line L501 (82.439, 17.2078) -> (82.439, 19.5228)
  line L502 (82.439, 19.5228) -> (81.6806, 19.1109)
  line L503 (81.6806, 19.1109) -> (81.5243, 19.4688)
  line L504 (81.5243, 19.4688) -> (82.5327, 20)
  line L505 (82.5327, 20) -> (82.9077, 20)
  line L506 (82.9077, 20) -> (82.9077, 17.2078)
  line L507 (82.9077, 17.2078) -> (83.615, 17.2078)
  line L508 (83.615, 17.2078) -> (83.615, 16.8158)
  spline S318 degree 2 poles (70.5167, 1.3696) (70.5167, 1.006) (70.3718, 0.4066) (70.0764, -0.0223) (69.6361, -0.2581) (69.3407, -0.2581) knots 0 0 0 1 2 3 4 4 4
  spline S319 degree 2 poles (69.3407, -0.2581) (69.0851, -0.2581) (68.6704, -0.0677) (68.3721, 0.3328) (68.213, 0.9463) (68.213, 1.3696) knots 0 0 0 1 2 3 4 4 4
  spline S320 degree 2 poles (68.213, 1.3696) (68.213, 1.7331) (68.3607, 2.3353) (68.6533, 2.7642) (69.0964, 3) (69.389, 3) knots 0 0 0 1 2 3 4 4 4
  spline S321 degree 2 poles (69.389, 3) (69.6447, 3) (70.0622, 2.8097) (70.3576, 2.4092) (70.5167, 1.7928) (70.5167, 1.3696) knots 0 0 0 1 2 3 4 4 4
  spline S322 degree 2 poles (70.0906, 1.3553) (70.0906, 1.4377) (70.0792, 1.5996) (70.0707, 1.6763) knots 0 0 0 1 2 2 2
  line L509 (70.0707, 1.6763) -> (68.73, 0.6822)
  spline S323 degree 2 poles (68.73, 0.6822) (68.7641, 0.5543) (68.8777, 0.3413) (69.0339, 0.1879) (69.2356, 0.1027) (69.3663, 0.1027) knots 0 0 0 1 2 3 4 4 4
  spline S324 degree 2 poles (69.3663, 0.1027) (69.531, 0.1027) (69.798, 0.2618) (69.9884, 0.5799) (70.0906, 1.0486) (70.0906, 1.3553) knots 0 0 0 1 2 3 4 4 4
  spline S325 degree 2 poles (68.6391, 1.3838) (68.6391, 1.3099) (68.642, 1.1594) (68.6476, 1.0883) knots 0 0 0 1 2 2 2
  line L510 (68.6476, 1.0883) -> (69.9912, 2.0797)
  spline S326 degree 2 poles (69.9912, 2.0797) (69.9543, 2.2047) (69.8435, 2.4092) (69.6873, 2.5569) (69.4884, 2.6393) (69.3663, 2.6393) knots 0 0 0 1 2 3 4 4 4
  spline S327 degree 2 poles (69.3663, 2.6393) (69.1987, 2.6393) (68.9317, 2.4802) (68.7414, 2.1621) (68.6391, 1.6934) (68.6391, 1.3838) knots 0 0 0 1 2 3 4 4 4
  line L511 (75.5557, 0.9066) -> (74.1042, 0.9066)
  line L512 (74.1042, 0.9066) -> (74.1042, 1.3042)
  line L513 (74.1042, 1.3042) -> (75.5557, 1.3042)
  line L514 (75.5557, 1.3042) -> (75.5557, 0.9066)
  line L515 (81.3475, -0.2154) -> (79.3563, -0.2154)
  line L516 (79.3563, -0.2154) -> (79.3563, 0.1765)
  line L517 (79.3563, 0.1765) -> (80.1716, 0.1765)
  line L518 (80.1716, 0.1765) -> (80.1716, 2.4916)
  line L519 (80.1716, 2.4916) -> (79.4131, 2.0797)
  line L520 (79.4131, 2.0797) -> (79.2569, 2.4376)
  line L521 (79.2569, 2.4376) -> (80.2653, 2.9688)
  line L522 (80.2653, 2.9688) -> (80.6402, 2.9688)
  line L523 (80.6402, 2.9688) -> (80.6402, 0.1765)
  line L524 (80.6402, 0.1765) -> (81.3475, 0.1765)
  line L525 (81.3475, 0.1765) -> (81.3475, -0.2154)
  spline S328 degree 2 poles (84.1795, 1.3696) (84.1795, 1.006) (84.0346, 0.4066) (83.7392, -0.0223) (83.2989, -0.2581) (83.0035, -0.2581) knots 0 0 0 1 2 3 4 4 4
  spline S329 degree 2 poles (83.0035, -0.2581) (82.7479, -0.2581) (82.3332, -0.0677) (82.0349, 0.3328) (81.8759, 0.9463) (81.8759, 1.3696) knots 0 0 0 1 2 3 4 4 4
  spline S330 degree 2 poles (81.8759, 1.3696) (81.8759, 1.7331) (82.0236, 2.3353) (82.3161, 2.7642) (82.7592, 3) (83.0518, 3) knots 0 0 0 1 2 3 4 4 4
  spline S331 degree 2 poles (83.0518, 3) (83.3075, 3) (83.725, 2.8097) (84.0204, 2.4092) (84.1795, 1.7928) (84.1795, 1.3696) knots 0 0 0 1 2 3 4 4 4
  spline S332 degree 2 poles (83.7534, 1.3553) (83.7534, 1.4377) (83.7421, 1.5996) (83.7335, 1.6763) knots 0 0 0 1 2 2 2
  line L526 (83.7335, 1.6763) -> (82.3928, 0.6822)
  spline S333 degree 2 poles (82.3928, 0.6822) (82.4269, 0.5543) (82.5405, 0.3413) (82.6968, 0.1879) (82.8984, 0.1027) (83.0291, 0.1027) knots 0 0 0 1 2 3 4 4 4
  spline S334 degree 2 poles (83.0291, 0.1027) (83.1938, 0.1027) (83.4609, 0.2618) (83.6512, 0.5799) (83.7534, 1.0486) (83.7534, 1.3553) knots 0 0 0 1 2 3 4 4 4
  spline S335 degree 2 poles (82.3019, 1.3838) (82.3019, 1.3099) (82.3048, 1.1594) (82.3104, 1.0883) knots 0 0 0 1 2 2 2
  line L527 (82.3104, 1.0883) -> (83.654, 2.0797)
  spline S336 degree 2 poles (83.654, 2.0797) (83.6171, 2.2047) (83.5063, 2.4092) (83.3501, 2.5569) (83.1512, 2.6393) (83.0291, 2.6393) knots 0 0 0 1 2 3 4 4 4
  spline S337 degree 2 poles (83.0291, 2.6393) (82.8615, 2.6393) (82.5945, 2.4802) (82.4042, 2.1621) (82.3019, 1.6934) (82.3019, 1.3838) knots 0 0 0 1 2 3 4 4 4
  line L528 (84.5601, 2.2189) -> (85.0402, 2.2189)
  line L529 (85.0402, 2.2189) -> (85.6338, 0.6083)
  line L530 (85.6338, 0.6083) -> (85.7645, 0.2135)
  line L531 (85.7645, 0.2135) -> (85.8952, 0.6168)
  line L532 (85.8952, 0.6168) -> (86.486, 2.2189)
  line L533 (86.486, 2.2189) -> (86.9518, 2.2189)
  line L534 (86.9518, 2.2189) -> (85.9946, -0.2154)
  line L535 (85.9946, -0.2154) -> (85.5117, -0.2154)
  line L536 (85.5117, -0.2154) -> (84.5601, 2.2189)
  spline S338 degree 2 poles (89.6816, 1.4036) (89.6816, 1.1764) (89.6105, 0.7588) (89.4572, 0.4009) (89.21, 0.1084) (88.8493, -0.1018) (88.3749, -0.2154) (88.071, -0.2154) knots 0 0 0 1 2 3 4 5 6 6 6
  line L537 (88.071, -0.2154) -> (87.3921, -0.2154)
  line L538 (87.3921, -0.2154) -> (87.3921, 2.9546)
  line L539 (87.3921, 2.9546) -> (88.2102, 2.9546)
  spline S339 degree 2 poles (88.2102, 2.9546) (88.9515, 2.9546) (89.6816, 2.1905) (89.6816, 1.4036) knots 0 0 0 1 2 2 2
  spline S340 degree 2 poles (89.2271, 1.3752) (89.2271, 1.7104) (89.1021, 2.1763) (88.8436, 2.4631) (88.4573, 2.591) (88.196, 2.591) knots 0 0 0 1 2 3 4 4 4
  line L540 (88.196, 2.591) -> (87.8239, 2.591)
  line L541 (87.8239, 2.591) -> (87.8239, 0.1595)
  line L542 (87.8239, 0.1595) -> (88.1448, 0.1595)
  spline S341 degree 2 poles (88.1448, 0.1595) (89.2271, 0.1595) (89.2271, 1.3752) knots 0 0 0 1 1 1
  spline S342 degree 2 poles (92.2749, -0.0961) (91.8943, -0.2552) (91.4767, -0.2552) knots 0 0 0 1 1 1
  spline S343 degree 2 poles (91.4767, -0.2552) (90.8064, -0.2552) (90.0849, 0.5486) (90.0849, 1.3355) knots 0 0 0 1 2 2 2
  spline S344 degree 2 poles (90.0849, 1.3355) (90.0849, 1.7161) (90.2837, 2.3325) (90.653, 2.7614) (91.1757, 2.9943) (91.5023, 2.9943) knots 0 0 0 1 2 3 4 4 4
  spline S345 degree 2 poles (91.5023, 2.9943) (91.721, 2.9943) (92.1017, 2.9176) (92.2749, 2.8409) knots 0 0 0 1 2 2 2
  line L543 (92.2749, 2.8409) -> (92.2749, 2.4177)
  spline S346 degree 2 poles (92.2749, 2.4177) (92.1017, 2.5114) (91.7324, 2.6109) (91.5165, 2.6109) knots 0 0 0 1 2 2 2
  spline S347 degree 2 poles (91.5165, 2.6109) (91.2921, 2.6109) (90.9314, 2.4433) (90.6786, 2.1251) (90.5422, 1.6678) (90.5422, 1.3724) knots 0 0 0 1 2 3 4 4 4
  spline S348 degree 2 poles (90.5422, 1.3724) (90.5422, 0.756) (91.0422, 0.1311) (91.525, 0.1311) knots 0 0 0 1 2 2 2
  spline S349 degree 2 poles (91.525, 0.1311) (91.7296, 0.1311) (92.1017, 0.2248) (92.2749, 0.31) knots 0 0 0 1 2 2 2
  line L544 (92.2749, 0.31) -> (92.2749, -0.0961)
  line L545 (120.7098, 16.7846) -> (120.2383, 16.7846)
  line L546 (120.2383, 16.7846) -> (120.0196, 17.4748)
  line L547 (120.0196, 17.4748) -> (118.6931, 17.4748)
  line L548 (118.6931, 17.4748) -> (118.4715, 16.7846)
  line L549 (118.4715, 16.7846) -> (118.0256, 16.7846)
  line L550 (118.0256, 16.7846) -> (119.0766, 19.9546)
  line L551 (119.0766, 19.9546) -> (119.6702, 19.9546)
  line L552 (119.6702, 19.9546) -> (120.7098, 16.7846)
  line L553 (119.8946, 17.8611) -> (119.3578, 19.5597)
  line L554 (119.3578, 19.5597) -> (118.8152, 17.8611)
  line L555 (118.8152, 17.8611) -> (119.8946, 17.8611)
  line L556 (121.8801, 19.591) -> (121.1501, 19.591)
  line L557 (121.1501, 19.591) -> (121.1501, 19.9546)
  line L558 (121.1501, 19.9546) -> (123.0476, 19.9546)
  line L559 (123.0476, 19.9546) -> (123.0476, 19.591)
  line L560 (123.0476, 19.591) -> (122.3176, 19.591)
  line L561 (122.3176, 19.591) -> (122.3176, 17.1538)
  line L562 (122.3176, 17.1538) -> (123.0476, 17.1538)
  line L563 (123.0476, 17.1538) -> (123.0476, 16.7846)
  line L564 (123.0476, 16.7846) -> (121.1501, 16.7846)
  line L565 (121.1501, 16.7846) -> (121.1501, 17.1538)
  line L566 (121.1501, 17.1538) -> (121.8801, 17.1538)
  line L567 (121.8801, 17.1538) -> (121.8801, 19.591)
  spline S350 degree 2 poles (128.5809, 17.7475) (128.5809, 17.5401) (128.4104, 17.1737) (128.0724, 16.8982) (127.5583, 16.7419) (127.2146, 16.7419) knots 0 0 0 1 2 3 4 4 4
  spline S351 degree 2 poles (127.2146, 16.7419) (127.0271, 16.7419) (126.726, 16.7675) (126.5954, 16.7874) knots 0 0 0 1 2 2 2
  line L568 (126.5954, 16.7874) -> (126.5954, 17.1652)
  spline S352 degree 2 poles (126.5954, 17.1652) (126.7459, 17.1368) (127.0811, 17.1084) (127.2544, 17.1084) knots 0 0 0 1 2 2 2
  spline S353 degree 2 poles (127.2544, 17.1084) (127.493, 17.1084) (127.831, 17.1936) (128.044, 17.3527) (128.1406, 17.5799) (128.1406, 17.7219) knots 0 0 0 1 2 3 4 4 4
  spline S354 degree 2 poles (128.1406, 17.7219) (128.1406, 17.8554) (128.0241, 18.0486) (127.8139, 18.1792) (127.5214, 18.2446) (127.3453, 18.2446) knots 0 0 0 1 2 3 4 4 4
  line L569 (127.3453, 18.2446) -> (126.9845, 18.2446)
  line L570 (126.9845, 18.2446) -> (126.9845, 18.5911)
  line L571 (126.9845, 18.5911) -> (127.3509, 18.5911)
  spline S355 degree 2 poles (127.3509, 18.5911) (127.493, 18.5911) (127.7287, 18.6678) (127.8935, 18.807) (127.9844, 19.0143) (127.9844, 19.145) knots 0 0 0 1 2 3 4 4 4
  spline S356 degree 2 poles (127.9844, 19.145) (127.9844, 19.4007) (127.6747, 19.6336) (127.3737, 19.6336) knots 0 0 0 1 2 2 2
  spline S357 degree 2 poles (127.3737, 19.6336) (127.2146, 19.6336) (126.8737, 19.5711) (126.6806, 19.5086) knots 0 0 0 1 2 2 2
  line L572 (126.6806, 19.5086) -> (126.6806, 19.8779)
  spline S358 degree 2 poles (126.6806, 19.8779) (126.7629, 19.9063) (126.9504, 19.9517) (127.1351, 19.983) (127.3197, 20) (127.4049, 20) knots 0 0 0 1 2 3 4 4 4
  spline S359 degree 2 poles (127.4049, 20) (127.6577, 20) (128.0412, 19.8921) (128.2968, 19.6875) (128.4275, 19.395) (128.4275, 19.2132) knots 0 0 0 1 2 3 4 4 4
  spline S360 degree 2 poles (128.4275, 19.2132) (128.4275, 18.9405) (128.1491, 18.5712) (127.9077, 18.4633) knots 0 0 0 1 2 2 2
  spline S361 degree 2 poles (127.9077, 18.4633) (128.0298, 18.4434) (128.2713, 18.3269) (128.4616, 18.1452) (128.5809, 17.898) (128.5809, 17.7475) knots 0 0 0 1 2 3 4 4 4
  spline S362 degree 2 poles (115.5167, 1.3696) (115.5167, 1.006) (115.3718, 0.4066) (115.0764, -0.0223) (114.6361, -0.2581) (114.3407, -0.2581) knots 0 0 0 1 2 3 4 4 4
  spline S363 degree 2 poles (114.3407, -0.2581) (114.0851, -0.2581) (113.6704, -0.0677) (113.3721, 0.3328) (113.213, 0.9463) (113.213, 1.3696) knots 0 0 0 1 2 3 4 4 4
  spline S364 degree 2 poles (113.213, 1.3696) (113.213, 1.7331) (113.3607, 2.3353) (113.6533, 2.7642) (114.0964, 3) (114.389, 3) knots 0 0 0 1 2 3 4 4 4
  spline S365 degree 2 poles (114.389, 3) (114.6447, 3) (115.0622, 2.8097) (115.3576, 2.4092) (115.5167, 1.7928) (115.5167, 1.3696) knots 0 0 0 1 2 3 4 4 4
  spline S366 degree 2 poles (115.0906, 1.3553) (115.0906, 1.4377) (115.0792, 1.5996) (115.0707, 1.6763) knots 0 0 0 1 2 2 2
  line L573 (115.0707, 1.6763) -> (113.73, 0.6822)
  spline S367 degree 2 poles (113.73, 0.6822) (113.7641, 0.5543) (113.8777, 0.3413) (114.0339, 0.1879) (114.2356, 0.1027) (114.3663, 0.1027) knots 0 0 0 1 2 3 4 4 4
  spline S368 degree 2 poles (114.3663, 0.1027) (114.531, 0.1027) (114.798, 0.2618) (114.9884, 0.5799) (115.0906, 1.0486) (115.0906, 1.3553) knots 0 0 0 1 2 3 4 4 4
  spline S369 degree 2 poles (113.6391, 1.3838) (113.6391, 1.3099) (113.642, 1.1594) (113.6476, 1.0883) knots 0 0 0 1 2 2 2
  line L574 (113.6476, 1.0883) -> (114.9912, 2.0797)
  spline S370 degree 2 poles (114.9912, 2.0797) (114.9543, 2.2047) (114.8435, 2.4092) (114.6873, 2.5569) (114.4884, 2.6393) (114.3663, 2.6393) knots 0 0 0 1 2 3 4 4 4
  spline S371 degree 2 poles (114.3663, 2.6393) (114.1987, 2.6393) (113.9317, 2.4802) (113.7414, 2.1621) (113.6391, 1.6934) (113.6391, 1.3838) knots 0 0 0 1 2 3 4 4 4
  line L575 (120.5557, 0.9066) -> (119.1042, 0.9066)
  line L576 (119.1042, 0.9066) -> (119.1042, 1.3042)
  line L577 (119.1042, 1.3042) -> (120.5557, 1.3042)
  line L578 (120.5557, 1.3042) -> (120.5557, 0.9066)
  line L579 (126.3759, -0.2154) -> (124.2882, -0.2154)
  line L580 (124.2882, -0.2154) -> (124.2882, 0.1623)
  line L581 (124.2882, 0.1623) -> (125.1062, 0.9776)
  spline S372 degree 2 poles (125.1062, 0.9776) (125.3079, 1.1764) (125.5607, 1.469) (125.6999, 1.7104) (125.7482, 1.9234) (125.7482, 2.0456) knots 0 0 0 1 2 3 4 4 4
  spline S373 degree 2 poles (125.7482, 2.0456) (125.7482, 2.1621) (125.6857, 2.3722) (125.555, 2.5342) (125.3448, 2.6251) (125.2, 2.6251) knots 0 0 0 1 2 3 4 4 4
  spline S374 degree 2 poles (125.2, 2.6251) (124.9983, 2.6251) (124.6688, 2.4461) (124.5324, 2.3012) knots 0 0 0 1 2 2 2
  line L582 (124.5324, 2.3012) -> (124.2995, 2.5824)
  spline S375 degree 2 poles (124.2995, 2.5824) (124.4785, 2.7699) (124.9472, 3) (125.2568, 3) knots 0 0 0 1 2 2 2
  spline S376 degree 2 poles (125.2568, 3) (125.467, 3) (125.8163, 2.875) (126.0663, 2.6364) (126.2055, 2.2927) (126.2055, 2.0768) knots 0 0 0 1 2 3 4 4 4
  spline S377 degree 2 poles (126.2055, 2.0768) (126.2055, 1.8922) (126.1089, 1.5826) (125.9129, 1.2758) (125.6147, 0.9463) (125.4102, 0.7475) knots 0 0 0 1 2 3 4 4 4
  line L583 (125.4102, 0.7475) -> (124.8364, 0.1879)
  line L584 (124.8364, 0.1879) -> (126.3759, 0.1879)
  line L585 (126.3759, 0.1879) -> (126.3759, -0.2154)
  spline S378 degree 2 poles (129.1795, 1.3696) (129.1795, 1.006) (129.0346, 0.4066) (128.7392, -0.0223) (128.2989, -0.2581) (128.0035, -0.2581) knots 0 0 0 1 2 3 4 4 4
  spline S379 degree 2 poles (128.0035, -0.2581) (127.7479, -0.2581) (127.3332, -0.0677) (127.0349, 0.3328) (126.8759, 0.9463) (126.8759, 1.3696) knots 0 0 0 1 2 3 4 4 4
  spline S380 degree 2 poles (126.8759, 1.3696) (126.8759, 1.7331) (127.0236, 2.3353) (127.3161, 2.7642) (127.7592, 3) (128.0518, 3) knots 0 0 0 1 2 3 4 4 4
  spline S381 degree 2 poles (128.0518, 3) (128.3075, 3) (128.725, 2.8097) (129.0204, 2.4092) (129.1795, 1.7928) (129.1795, 1.3696) knots 0 0 0 1 2 3 4 4 4